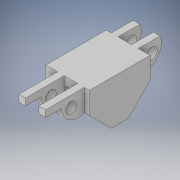
# Autodesk Inventor part: finger_joins
Saved by Autodesk Inventor 2019 (Build 230136000, 136)
## iProperties
Created: 2018-09-13
Part Number: finger_joins
Material: Generic
Document SubType Name: Modeling
Designer: jerem
Density: 1 g/cm^3
Appearance: Default
Author: jerem
Autodesk Inventor part; units mm, degrees
ref_plane "YZ Plane" through (0, 0, 0) normal (1, 0, 0) x (0, 1, 0)
ref_plane "XZ Plane" through (0, 0, 0) normal (0, 1, 0) x (-1, 0, 0)
ref_plane "XY Plane" through (0, 0, 0) normal (0, 0, 1) x (1, 0, 0)
sketch "Sketch7" plane through (0, 0, 0) normal (1, 0, 0) x (0, 1, 0)
  line L0 (-2.6, 0) -> (15.6, 0) projected
  line L1 (0, -24.701) -> (0, 24.701) projected
  line L2 (0, 2.5) -> (0, -2.5)
  line L3 (13, 15.5) -> (13, 0)
  line L4 (0, 2.5) -> (6.5, 9)
  line L5 (0, 2.5) -> (9.1924, 2.5) construction
  arc A0 (13, 15.5) -> (6.5, 9) centre (11.1419, 10.8581) ccw
  circle A1 centre (9.75, 13) radius 1.625
  line L6 (13, -15.5) -> (13, 0)
  line L7 (0, -2.5) -> (6.5, -9)
  arc A2 (6.5, -9) -> (13, -15.5) centre (11.1419, -10.8581) ccw
  circle A3 centre (9.75, -13) radius 1.625
  point P0 (0, 0)
  dimension "d64" = 5
  dimension "d65" = 2.5
  dimension "d66" = 45
  dimension "d67" = 6.5
  dimension "d68" = 13
  dimension "d69" = 15.5
  dimension "d70" = 5
  dimension "d71" = 3.25
  dimension "d74" = 3.25
  dimension "d103" = 2.5
  constraints: 12 end point, 4 centre point, 4 point on circle, 4 symmetric about line, 2 vertical, 1 collinear, 1 equal length, 1 horizontal, 1 perpendicular, 1 point on line, 2 other
  measures "d64" distance of L2.start L2.end
  measures "d65" distance from line of L2.start L0
  measures "d66" angle of L5 L4
  measures "d67" horizontal distance of L2.start L4.end
  measures "d68" distance between parallel lines of L3 L2
  measures "d69" distance of L3.start L3.end
  measures "d70" radius of A0
  measures "d71" diameter of A1
  measures "d74" distance from line of L3 A1.centre
  measures "d103" vertical distance of A1.centre L3.start
extrude "Extrusion5" add sketch "Sketch7" along normal mid plane 13
sketch "Sketch8" plane through (-6.5, 13, 15.5) normal (0, 1, 0) x (1, 0, 0)
  line L0 (0, 6.5) -> (13, 6.5) projected
  line L1 (11.5, 6.5) -> (13, 6.5)
  line L2 (13, 6.5) -> (13, -0.5)
  line L3 (13, -0.5) -> (11.5, -0.5)
  line L4 (11.5, -0.5) -> (11.5, 6.5)
  line L5 (13, 31) -> (13, 0) projected
  line L6 (5.5, 6.5) -> (9.5, 6.5)
  line L7 (9.5, 6.5) -> (9.5, -0.5)
  line L8 (9.5, -0.5) -> (5.5, -0.5)
  line L9 (5.5, -0.5) -> (5.5, 6.5)
  line L10 (0, 6.5) -> (3.5, 6.5)
  line L11 (3.5, 6.5) -> (3.5, -0.5)
  line L12 (3.5, -0.5) -> (0, -0.5)
  line L13 (0, -0.5) -> (0, 6.5)
  line L14 (0, 0) -> (0, 31) projected
  point P0 (6.5, 15.5)
  dimension "d77" = 1.5
  dimension "d78" = 7
  dimension "d79" = 4
  dimension "d80" = 7
  dimension "d81" = 2
  dimension "d83" = 7
  dimension "d101" = 2
  constraints: 24 end point, 6 parallel, 5 collinear, 3 horizontal, 3 perpendicular
  measures "d77" distance of L2.end L3.end
  measures "d78" distance of L1.end L2.end
  measures "d79" distance of L7.end L8.end
  measures "d80" distance of L6.end L7.end
  measures "d81" distance between parallel lines of L7 L4
  measures "d83" distance of L10.end L11.end
  measures "d101" distance between parallel lines of L11 L9
extrude "Extrusion6" cut sketch "Sketch8" against normal blind 10
sketch "Sketch9" plane through (-6.5, 13, -15.5) normal (0, 1, 0) x (1, 0, 0)
  line L0 (0, -6.5) -> (13, -6.5) projected
  line L1 (1.5, -6.5) -> (0, -6.5)
  line L2 (0, -6.5) -> (0, 0.5)
  line L3 (0, 0.5) -> (1.5, 0.5)
  line L4 (1.5, 0.5) -> (1.5, -6.5)
  line L5 (0, -24.5) -> (0, 0) projected
  line L6 (7.5, -6.5) -> (3.5, -6.5)
  line L7 (3.5, -6.5) -> (3.5, 0.5)
  line L8 (3.5, 0.5) -> (7.5, 0.5)
  line L9 (7.5, 0.5) -> (7.5, -6.5)
  line L10 (13, -6.5) -> (9.5, -6.5)
  line L11 (9.5, -6.5) -> (9.5, 0.5)
  line L12 (9.5, 0.5) -> (13, 0.5)
  line L13 (13, 0.5) -> (13, -6.5)
  line L14 (13, 0) -> (13, -24.5) projected
  point P0 (6.5, -15.5)
  dimension "d86" = 1.5
  dimension "d87" = 7
  dimension "d88" = 4
  dimension "d89" = 7
  dimension "d90" = 2
  dimension "d92" = 7
  dimension "d102" = 2
  constraints: 24 end point, 6 parallel, 5 collinear, 3 horizontal, 3 perpendicular
  measures "d86" distance of L2.end L3.end
  measures "d87" distance of L1.end L2.end
  measures "d88" distance of L7.end L8.end
  measures "d89" distance of L6.end L7.end
  measures "d90" distance between parallel lines of L4 L7
  measures "d92" distance of L10.end L11.end
  measures "d102" distance between parallel lines of L11 L9
extrude "Extrusion7" cut sketch "Sketch9" against normal blind 10
sketch "Sketch10" plane through (1, 13, -9) normal (0, 0, -1) x (-1, 0, 0)
  line L0 (1, -15.6) -> (1, 2.6) projected
  line L1 (7.5, -13) -> (-5.5, -13) projected
  circle A0 centre (1, -3) radius 0.75
  line L2 (0, 0) -> (4, 0) projected
  circle A1 centre (1, -10) radius 0.75
  point P0 (1, -13)
  dimension "d95" = 1.5
  dimension "d96" = 3
  dimension "d97" = 1.5
  dimension "d98" = 3
  constraints: 2 centre point, 2 point on line
  measures "d95" diameter of A0
  measures "d96" distance from line of L2 A0.centre
  measures "d97" diameter of A1
  measures "d98" distance from line of L1 A1.centre
extrude "Extrusion8" cut sketch "Sketch10" against normal blind 20
sketch "Sketch13" plane through (5, 13, 15.5) normal (1, 0, 0) x (0, 0, -1)
  line L0 (-5, 0) -> (0, 0)
  line L1 (0, 0) -> (0, -2)
  line L2 (0, -2) -> (-5, -2)
  line L3 (-5, -2) -> (-5, 0)
  line L4 (0, 0) -> (6.5, 0) projected
  point P0 (15.5, -13)
  dimension "d112" = 5
  dimension "d113" = 2
  constraints: 8 end point, 2 parallel, 1 collinear, 1 horizontal, 1 perpendicular
  measures "d112" distance of L1.end L2.end
  measures "d113" distance of L0.end L1.end
extrude "Extrusion11" add sketch "Sketch13" against normal blind 2
sketch "Sketch14" plane through (-3, 13, 9) normal (-1, 0, 0) x (0, 0, 1)
  line L0 (6.5, 0) -> (0, 0) projected
  line L1 (6.5, 0) -> (11.5, 0)
  line L2 (11.5, 0) -> (11.5, -2)
  line L3 (11.5, -2) -> (6.5, -2)
  line L4 (6.5, -2) -> (6.5, 0)
  point P0 (-9, -13)
  dimension "d116" = 5
  dimension "d117" = 2
  constraints: 8 end point, 2 parallel, 1 collinear, 1 horizontal, 1 perpendicular
  measures "d116" distance of L2.end L3.end
  measures "d117" distance of L1.end L2.end
extrude "Extrusion12" add sketch "Sketch14" against normal blind 2
body "Solid2"
